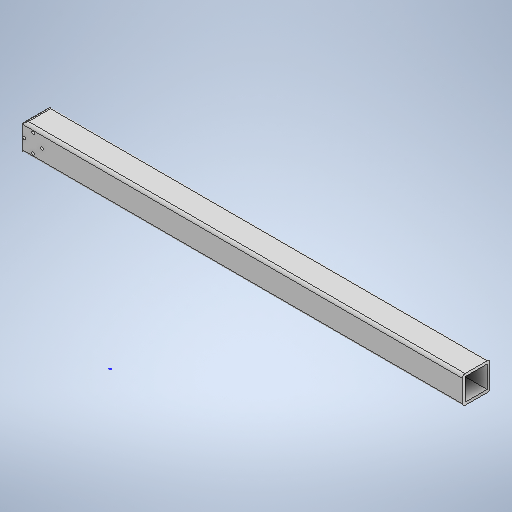
# Autodesk Inventor part: rockerpivotarm
Saved by Autodesk Inventor 2025.4 (Build 294407000, 407)
## iProperties
Created: 2026-03-21
Part Number: rockerpivotarm
Material: Generic
Document SubType Name: Modeling
Designer: hp
Density: 1 g/cm^3
Appearance: Default
Author: hp
Autodesk Inventor part; units mm, degrees
ref_plane "YZ Plane" through (0, 0, 0) normal (1, 0, 0) x (0, 1, 0)
ref_plane "XZ Plane" through (0, 0, 0) normal (0, 1, 0) x (-1, 0, 0)
ref_plane "XY Plane" through (0, 0, 0) normal (0, 0, 1) x (1, 0, 0)
sketch "Sketch1" plane through (0, 0, 0) normal (1, 0, 0) x (0, 1, 0)
  line L0 (2, 0) -> (18, 0)
  line L1 (20, -2) -> (20, -18)
  line L2 (18, -20) -> (2, -20)
  line L3 (0, -18) -> (0, -2)
  line L4 (18, -18) -> (18, -2)
  line L5 (18, -2) -> (2, -2)
  line L6 (2, -2) -> (2, -18)
  line L7 (2, -18) -> (18, -18)
  arc A0 (20, -2) -> (18, 0) centre (18, -2) ccw
  arc A1 (18, -20) -> (20, -18) centre (18, -18) ccw
  arc A2 (0, -18) -> (2, -20) centre (2, -18) ccw
  arc A3 (2, 0) -> (0, -2) centre (2, -2) ccw
  point P0 (0, 0)
  point P1 (20, -20)
  point P2 (20, 0)
  point P3 (0, -20)
  dimension "d0" = 20
  dimension "d1" = 20
  dimension "d2" = 2
  dimension "d5" = 2
  constraints: 16 end point, 8 point on circle, 8 point on line, 8 tangent, 4 centre point, 4 parallel, 3 equal radius, 2 perpendicular, 1 horizontal, 3 other
  measures "d0" distance of point (20, -20) point (0, -20)
  measures "d1" distance of point (20, 0) point (20, -20)
  measures "d2" distance between parallel lines of L1 L4
  measures "d5" radius of A0
extrude "Extrusion1" add sketch "Sketch1" along normal blind 319
sketch "Sketch2" plane through (0, 0, -18) normal (0, -1, 0) x (1, 0, 0)
  line L0 (0, 16) -> (0, 0) projected
  line L1 (0, 0) -> (319, 0) projected
  point P0 (0, 18)
  point P1 (16, 8)
  dimension "d6" = 16
  dimension "d7" = 8
  measures "d6" distance from line of point (16, 8) L0
  measures "d7" distance from line of point (16, 8) L1
hole "Hole1" at (16, 0, -10) direction (0, 1, 0) diameter 2.45 depth 2
sketch "Sketch4" plane through (0, 2, -20) normal (0, 0, -1) x (-1, 0, 0)
  line L0 (0, 0) -> (0, 16) projected
  line L1 (0, 16) -> (-319, 16) projected
  line L2 (0, 0) -> (-16, 0)
  line L3 (-16, 0) -> (-16, 16)
  line L4 (-16, 16) -> (0, 16)
  line L5 (0, 16) -> (0, 0)
  circle A0 centre (-8, 8) radius 8
  circle A1 centre (-8, 8) radius 5
  circle A2 centre (-8, 8) radius 6.5
  line L6 (0, 18) -> (-319, 18) projected
  line L7 (-2.6429, 18) -> (0, 16.4741)
  line L8 (-2.6429, 18) -> (-0.6491, 18) construction
  line L9 (0, 18) -> (0, 16) projected
  point P0 (0, -2)
  point P1 (-8, 1.5)
  point P2 (-1.5, 8)
  point P3 (-8, 14.5)
  point P4 (-14.5, 8)
  dimension "d21" = 10
  dimension "d22" = 13
  dimension "d30" = 30
  dimension "d33" = 2.6429
  constraints: 12 end point, 4 point on circle, 3 centre point, 3 point on line, 2 coincident, 2 horizontal, 2 parallel, 1 perpendicular, 1 tangent
  measures "d21" diameter of A1
  measures "d22" diameter of A2
  measures "d30" angle of L7 L8
  measures "d33" distance of L6.start L7.start
extrude "Extrusion3" cut sketch "Sketch4" against normal up to surface (2 mm away) contours A1
hole "Hole2" at (8, 3.5, -20) at (1.5, 10, -20) at (14.5, 10, -20) at (8, 16.5, -20) direction (0, 0, 1) diameter 2 end through all
extrude "Extrusion4" cut sketch "Sketch4" against normal up to next contours L7 L6 L9
body "Solid1"
